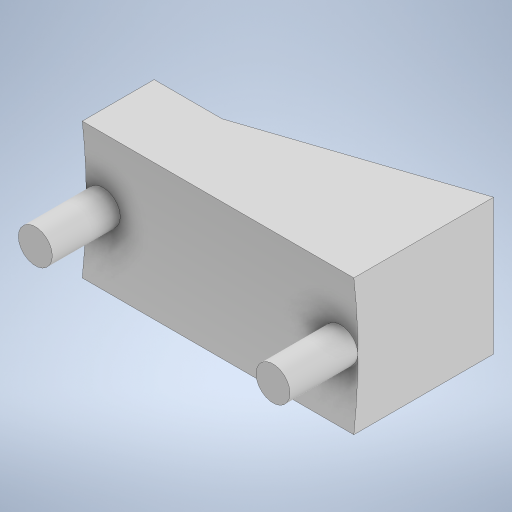
# Autodesk Inventor part: last
Saved by Autodesk Inventor 2023 (Build 270158000, 158)
## iProperties
Created: 2023-11-07
Part Number: last
Material: Generic
Document SubType Name: Modeling
Designer: Rahul
Density: 1 g/cm^3
Appearance: Default
Author: Rahul
Autodesk Inventor part; units mm, degrees
ref_plane "YZ Plane" through (0, 0, 0) normal (1, 0, 0) x (0, 1, 0)
ref_plane "XZ Plane" through (0, 0, 0) normal (0, 1, 0) x (-1, 0, 0)
sketch "Sketch1" plane through (0, 0, 0) normal (0, 1, 0) x (-1, 0, 0)
  line L0 (0, 0) -> (0, -2)
  line L1 (0, -2) -> (3, -1)
  line L2 (3, -1) -> (4, -1)
  line L3 (4, -1) -> (4, 0)
  line L4 (4, 0) -> (0, 0)
  dimension "d0" = 1
  dimension "d1" = 2
  dimension "d2" = 1
  dimension "d3" = 4
  constraints: 10 end point, 3 perpendicular, 1 vertical
  measures "d0" distance of L2.end L3.end
  measures "d1" distance of L0.start L0.end
  measures "d2" distance of L1.end L2.end
  measures "d3" distance between parallel lines of L0 L3
extrude "Extrusion1" add sketch "Sketch1" along normal blind 2
sketch "Sketch2" plane through (-4, 0, -1) normal (-1, 0, 0) x (0, 0, 1)
  line L0 (0, 0) -> (1, 0) projected
  line L1 (1, 0) -> (1, 1)
  line L2 (1, 0) -> (1, 2) projected
  line L3 (1, 1) -> (9.5, 1)
  line L4 (1, 1) -> (9.5, 1) construction
  arc A0 (1, 1) -> (1.059, 0) centre (9.5, 1) ccw
  arc A1 (1.059, 2) -> (1, 1) centre (9.5, 1) ccw
  line L5 (1.059, 0) -> (1, 0)
  line L6 (0, 2) -> (1, 2) projected
  line L7 (1.059, 2) -> (1, 2)
  line L8 (1, 0) -> (1, 2)
  dimension "d6" = 1
  dimension "d7" = 8.5
  dimension "d8" = 0
  constraints: 12 end point, 4 horizontal, 4 point on circle, 2 centre point, 2 collinear, 1 coincident, 1 midpoint, 1 symmetric about line, 1 other
  measures "d6" distance of L0.end L1.end
  measures "d7" distance of L1.end L3.end
  measures "d8" distance between parallel lines of L3 L4
extrude "Extrusion2" add sketch "Sketch2" against normal up to surface (4 mm away)
ref_plane "Work Plane1" through (-4, 1, 0) normal (0, 0, 1) x (1, 0, 0)
sketch "Sketch3" plane through (-4, 1, 0) normal (0, 0, 1) x (1, 0, 0)
  circle A0 centre (3.75, 0) radius 0.25
  line L0 (4, -1) -> (4, 1) projected
  dimension "d11" = 0.5
  constraints: 1 centre point, 1 tangent
  measures "d11" diameter of A0
extrude "Extrusion3" add sketch "Sketch3" along normal blind 1
sketch "Sketch4" plane through (-4, 1, 0) normal (0, 0, 1) x (1, 0, 0)
  circle A0 centre (0.25, 0) radius 0.25
  line L0 (0, -1) -> (0, 1) projected
  circle A1 centre (3.75, 0) radius 0.25 projected
  point P0 (4, -1)
  point P1 (3.75, 0.25)
  dimension "d14" = 0.5
  constraints: 1 centre point, 1 tangent, 1 vertical alignment, 1 other
  measures "d14" diameter of A0
extrude "Extrusion4" add sketch "Sketch4" along normal up to surface (1 mm away) contours A0
body "Solid1"
